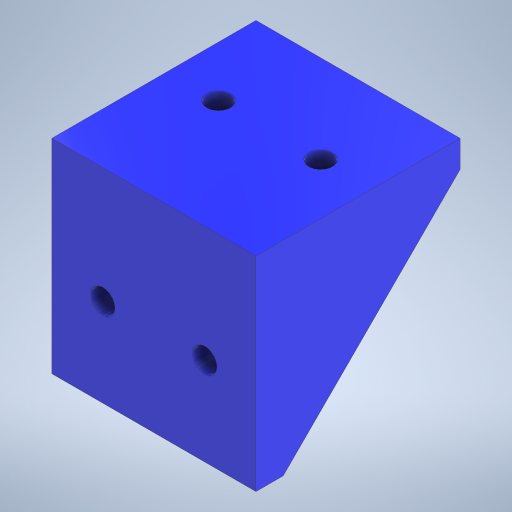
# Autodesk Inventor part: Union
Saved by Autodesk Inventor 2024 (Build 280153000, 153)
## iProperties
Created: 2023-07-05
Part Number: Union
Material: Genérico
Document SubType Name: Modeling
Designer: sergi
Density: 1 g/cm^3
Appearance: Valor por defecto
Author: sergi
Autodesk Inventor part; units mm, degrees
ref_plane "YZ Plane" through (0, 0, 0) normal (1, 0, 0) x (0, 1, 0)
ref_plane "XZ Plane" through (0, 0, 0) normal (0, 1, 0) x (-1, 0, 0)
ref_plane "XY Plane" through (0, 0, 0) normal (0, 0, 1) x (1, 0, 0)
sketch "Boceto1" plane through (0, 0, 0) normal (0, 0, 1) x (1, 0, 0)
  line L0 (0, 0) -> (30, 0)
  line L1 (30, 0) -> (30, -30)
  line L2 (30, -30) -> (0, -30)
  line L3 (0, -30) -> (0, 0)
  dimension "d0" = 30
  dimension "d1" = 30
  constraints: 8 end point, 2 parallel, 1 horizontal, 1 perpendicular
  measures "d0" distance of L1.end L2.end
  measures "d1" distance of L0.end L1.end
extrude "Extrusión1" add sketch "Boceto1" along normal blind 4
sketch "Boceto2" plane through (0, 0, 0) normal (0, 1, 0) x (1, 0, 0)
  line L0 (30, -4) -> (0, -4) projected
  line L1 (0, -4) -> (30, -4)
  line L2 (30, -4) -> (30, 26)
  line L3 (30, 26) -> (0, 26)
  line L4 (0, 26) -> (0, -4)
  point P0 (0, 0)
  dimension "d4" = 30
  constraints: 8 end point, 2 parallel, 1 horizontal, 1 perpendicular
  measures "d4" distance of L2.end L1.end
extrude "Extrusión2" add sketch "Boceto2" against normal blind 4
sketch "Boceto3" plane through (0, 0, 0) normal (0, 0, -1) x (-1, 0, 0)
  line L0 (0, -4) -> (-30, -4) projected
  line L1 (-30, -30) -> (-30, -4) projected
  line L2 (0, -30) -> (-30, -30) projected
  line L3 (0, -4) -> (0, -30) projected
  line L4 (0, -30) -> (-30, -30) projected
  line L5 (-15, -30) -> (-15, -4)
  line L6 (0, -4) -> (0, -30) projected
  line L7 (0, -17) -> (-30, -17)
  line L8 (-30, -17) -> (-22.5, -17)
  circle A0 centre (-22.5, -17) radius 3
  line L9 (0, -17) -> (-7.5, -17)
  circle A1 centre (-7.5, -17) radius 3
  point P0 (0, 0)
  dimension "d7" = 7.5
  dimension "d8" = 6
  dimension "d9" = 7.5
  dimension "d10" = 6
  constraints: 8 end point, 4 midpoint, 2 centre point, 2 coincident, 2 point on line
  measures "d7" distance of L7.end L8.end
  measures "d8" diameter of A0
  measures "d9" distance of L7.start L9.end
  measures "d10" diameter of A1
hole "Agujero1" at (22.5, -17, 0) at (7.5, -17, 0) direction (0, 0, 1) diameter 3.5 end through all countersink diameter 6 countersink angle 90
sketch "Boceto4" plane through (0, 0, 0) normal (0, 0, -1) x (-1, 0, 0)
  line L0 (0, -30) -> (-30, -30) projected
  line L1 (0, 0) -> (-3, 0)
  line L2 (-3, 0) -> (-3, -30)
  line L3 (-3, -30) -> (0, -30)
  line L4 (0, -30) -> (0, 0)
  line L5 (-30, -30) -> (-27, -30)
  line L6 (-27, -30) -> (-27, 0)
  line L7 (-27, 0) -> (-30, 0)
  line L8 (-30, 0) -> (-30, -30)
  dimension "d18" = 3
  dimension "d19" = 3
  constraints: 16 end point, 4 parallel, 2 horizontal, 2 perpendicular, 2 point on line
  measures "d18" distance of L3.end L2.end
  measures "d19" distance of L7.end L6.end
extrude "Extrusión3" add sketch "Boceto4" along normal up to surface (26 mm away)
sketch "Boceto5" plane through (30, -30, 4) normal (1, 0, 0) x (0, 0, -1)
  line L0 (30, 26) -> (4, 0)
  line L1 (30, 30) -> (0, 30) projected
  line L2 (0, 0) -> (0, 30) projected
  line L3 (30, 0) -> (0, 0) projected
  line L4 (30, 30) -> (30, 0) projected
  point P0 (4, 30)
  constraints: 2 end point
extrude "Extrusión4" cut sketch "Boceto5" against normal through all contours L4 L3 L0
sketch "Boceto8" plane through (0, -4, 0) normal (0, -1, 0) x (1, 0, 0)
  line L0 (3, 0) -> (3, -26) projected
  line L1 (3, -26) -> (27, -26) projected
  line L2 (27, -26) -> (27, 0) projected
  line L3 (3, 0) -> (27, 0) projected
  line L4 (25.5, 0) -> (19.5, 0) projected
  line L5 (10.5, 0) -> (4.5, 0) projected
  line L6 (22.5, 0) -> (22.5, -26)
  line L7 (7.5, 0) -> (7.5, -26)
  line L8 (3, -26) -> (27, -26) projected
  line L9 (27, -26) -> (27, 0) projected
  line L10 (27, -13) -> (3, -13)
  circle A0 centre (22.5, -13) radius 1.75
  circle A1 centre (7.5, -13) radius 1.75
  point P0 (0, 0)
  dimension "d25" = 3.5
  dimension "d26" = 3.5
  constraints: 6 end point, 6 midpoint, 4 point on line, 2 centre point, 1 parallel, 1 perpendicular
  measures "d25" diameter of A0
  measures "d26" diameter of A1
hole "Agujero2" at (22.5, -4, -13) at (7.5, -4, -13) direction (0, 1, 0) diameter 3.5 end through all countersink diameter 6 countersink angle 90
